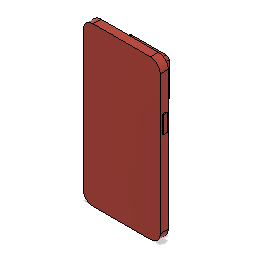
IPHONE_14Plus (PENDING CHECK) v4 (Autodesk Fusion 360 design; units mm, degrees)
Autodesk Fusion 360 part; units mm, degrees
sketch "Sketch1" plane through (0, 0, 0) normal (0, 0, 1) x (1, 0, 0)
  line L0 (39.05, 80.4) -> (-39.05, 80.4)
  line L1 (-39.05, 80.4) -> (-39.05, -80.4)
  line L2 (-39.05, -80.4) -> (39.05, -80.4)
  line L3 (39.05, -80.4) -> (39.05, 80.4)
  line L4 (39.05, 80.4) -> (-39.05, -80.4) construction
  line L5 (-39.05, 80.4) -> (39.05, -80.4) construction
  dimension "d1" = 78.1
  dimension "d2" = 160.8
  constraint horizontal L0
  constraint perpendicular L0 L1
  constraint parallel L0 L2
  constraint parallel L1 L3
  constraint coincident L4 origin
  constraint coincident L5 origin
  measures "d1" distance of L1.end L2.end
  measures "d2" distance of L0.end L1.end
extrude "Extrude1" add sketch "Sketch1" along normal blind 7.8 makes body 1
fillet "Fillet1" radius 10 4 edges at (-39.05, 80.4, 3.9) (39.05, 80.4, 3.9) (39.05, -80.4, 3.9) (-39.05, -80.4, 3.9) on bodies 1
sketch "Sketch3" plane through (0, 0, 0) normal (0, 0, -1) x (1, 0, 0)
  line L0 (-5.7, -37.375) -> (35.3, -37.375)
  line L1 (35.3, -37.375) -> (35.3, -77.375)
  line L2 (35.3, -77.375) -> (-5.7, -77.375)
  line L3 (-5.7, -77.375) -> (-5.7, -37.375)
  line L4 (-5.7, -37.375) -> (35.3, -77.375) construction
  line L5 (35.3, -37.375) -> (-5.7, -77.375) construction
  line L6 (-28.8, -80.375) -> (28.8, -80.375)
  line L7 (38.8, -70.375) -> (38.8, 70.375)
  arc A0 (-28.8, 80.375) -> (-38.8, 70.375) centre (-28.8, 70.375) ccw
  line L8 (-28.8, 80.375) -> (28.8, 80.375)
  arc A1 (38.8, 70.375) -> (28.8, 80.375) centre (28.8, 70.375) ccw
  line L9 (38.8, 70.375) -> (38.8, -70.375)
  arc A2 (28.8, -80.375) -> (38.8, -70.375) centre (28.8, -70.375) ccw
  line L10 (28.8, -80.375) -> (-28.8, -80.375)
  arc A3 (-38.8, -70.375) -> (-28.8, -80.375) centre (-28.8, -70.375) ccw
  line L11 (-38.8, -70.375) -> (-38.8, 70.375)
  arc A4 (-29.05, 80.4) -> (-39.05, 70.4) centre (-29.05, 70.4) ccw
  line L12 (-39.05, 70.4) -> (-39.05, -70.4)
  arc A5 (-39.05, -70.4) -> (-29.05, -80.4) centre (-29.05, -70.4) ccw
  line L13 (-29.05, -80.4) -> (29.05, -80.4)
  arc A6 (29.05, -80.4) -> (39.05, -70.4) centre (29.05, -70.4) ccw
  line L14 (39.05, -70.4) -> (39.05, 70.4)
  arc A7 (39.05, 70.4) -> (29.05, 80.4) centre (29.05, 70.4) ccw
  line L15 (29.05, 80.4) -> (-29.05, 80.4)
  point P0 (14.8, -57.375)
  dimension "d9" = 41
  dimension "d10" = 40
  dimension "d18" = 3
  dimension "d19" = 3.5
  constraint horizontal L0
  constraint perpendicular L0 L1
  constraint parallel L0 L2
  constraint parallel L1 L3
  constraint coincident L4 P0
  constraint coincident L5 P0
  measures "d9" distance of L0.start L0.end
  measures "d10" distance of L0.start L2.end
  measures "d18" distance of L2 L6
  measures "d19" distance of L1 L9
extrude "Extrude2" add sketch "Sketch3" along normal blind 4.5 contours L0 L1 L2 L3 bodies 1
fillet "Fillet2" radius 3 4 edges at (35.3, 77.375, -2.25) (35.3, 37.375, -2.25) (-5.7, 77.375, -2.25) (-5.7, 37.375, -2.25) on bodies 1
sketch "Sketch4" plane through (39.05, 0, 0) normal (1, 0, 0) x (0, 0, -1)
  line L0 (-7.8, -70.4) -> (0, -70.4)
  line L1 (0, -70.4) -> (0, 70.4)
  line L2 (0, 70.4) -> (-7.8, 70.4)
  line L3 (-7.8, 70.4) -> (-7.8, -70.4)
  line L4 (4.5, 40.375) -> (4.5, 37.375)
  line L5 (4.5, 37.375) -> (0, 37.375)
  line L6 (4.5, 40.375) -> (4.5, 74.375)
  line L7 (4.5, 77.375) -> (4.5, 74.375)
  line L8 (0, 77.375) -> (4.5, 77.375)
  line L9 (-7.8, -80.4) -> (-7.8, -70.4)
  line L10 (0, -70.4) -> (0, -80.4)
  line L11 (0, -80.4) -> (-7.8, -80.4)
  line L12 (0, 37.375) -> (0, -70.4)
  line L13 (0, 80.4) -> (0, 77.375)
  line L14 (-7.8, 80.4) -> (0, 80.4)
  line L15 (-7.8, 70.4) -> (-7.8, 80.4)
  line L16 (-7.8, 70.4) -> (-7.8, -70.4)
  line L17 (-3.9, 70.4) -> (-3.9, -70.4) construction
  line L18 (-1.9, 16.2) -> (-5.9, 16.2)
  line L19 (-5.9, 16.2) -> (-5.9, 33.9)
  line L20 (-5.9, 33.9) -> (-1.9, 33.9)
  line L21 (-1.9, 33.9) -> (-1.9, 16.2)
  line L22 (-1.9, 16.2) -> (-5.9, 33.9) construction
  line L23 (-5.9, 16.2) -> (-1.9, 33.9) construction
  point P0 (-3.9, 25.05)
  dimension "d20" = 4
  dimension "d21" = 17.7
  dimension "d22" = 46.5
  constraint midpoint L2 L17.start
  constraint midpoint L0 L17.end
  constraint horizontal L18
  constraint perpendicular L18 L19
  constraint parallel L18 L20
  constraint parallel L19 L21
  constraint coincident L22 P0
  constraint coincident L23 P0
  constraint coincident L17 P0
  measures "d20" distance of L18.start L18.end
  measures "d21" distance of L18.start L20.end
  measures "d22" distance of L14 L20
extrude "Extrude3" add sketch "Sketch4" along normal blind 1 contours L18 L19 L20 L21 bodies 1
sketch "Sketch5" plane through (-39.05, 0, 0) normal (-1, 0, 0) x (0, 0, 1)
  line L0 (0, -70.4) -> (7.8, -70.4)
  line L1 (7.8, -70.4) -> (7.8, 70.4)
  line L2 (7.8, 70.4) -> (0, 70.4)
  line L3 (0, 70.4) -> (0, -70.4)
  line L4 (-4.5, 74.375) -> (-4.5, 77.375)
  line L5 (-4.5, 74.375) -> (-4.5, 40.375)
  line L6 (-4.5, 37.375) -> (-4.5, 40.375)
  line L7 (0, 37.375) -> (-4.5, 37.375)
  line L8 (-4.5, 77.375) -> (0, 77.375)
  line L9 (7.8, -80.4) -> (0, -80.4)
  line L10 (0, 77.375) -> (0, 80.4)
  line L11 (0, -70.4) -> (0, 37.375)
  line L12 (0, -80.4) -> (0, -70.4)
  line L13 (7.8, -70.4) -> (7.8, -80.4)
  line L14 (7.8, -70.4) -> (7.8, 70.4)
  line L15 (7.8, 80.4) -> (7.8, 70.4)
  line L16 (0, 80.4) -> (7.8, 80.4)
  line L17 (3.9, 70.4) -> (3.9, -70.4) construction
  line L18 (5.225, 30.45) -> (2.575, 30.45)
  line L19 (2.575, 30.45) -> (2.575, 41.65)
  line L20 (2.575, 41.65) -> (5.225, 41.65)
  line L21 (5.225, 41.65) -> (5.225, 30.45)
  line L22 (5.225, 30.45) -> (2.575, 41.65) construction
  line L23 (2.575, 30.45) -> (5.225, 41.65) construction
  line L24 (0, 28.95) -> (7.8, 28.95) construction
  line L25 (2.575, 27.45) -> (2.575, 16.25)
  line L26 (2.575, 16.25) -> (5.225, 16.25)
  line L27 (5.225, 27.45) -> (2.575, 27.45)
  line L28 (5.225, 16.25) -> (5.225, 27.45)
  point P0 (3.9, 36.05)
  dimension "d25" = 1.5
  dimension "d26" = 11.2
  dimension "d27" = 2.65
  dimension "d28" = 38.75
  constraint midpoint L2 L17.start
  constraint midpoint L0 L17.end
  constraint horizontal L18
  constraint perpendicular L18 L19
  constraint parallel L18 L20
  constraint parallel L19 L21
  constraint coincident L22 P0
  constraint coincident L23 P0
  constraint coincident L17 P0
  constraint coincident L11 L24.start
  constraint coincident L14 L24.end
  constraint perpendicular L14 L24
  constraint symmetric L18.start L24 L27.start
  constraint symmetric L18.end L24 L25.start
  constraint symmetric L19.end L24 L25.end
  constraint symmetric L20.end L24 L26.end
  measures "d25" distance of L18 L24
  measures "d26" distance of L18.start L20.end
  measures "d27" distance of L18.start L18.end
  measures "d28" distance of L16 L20
extrude "Extrude4" add sketch "Sketch5" along normal blind 1 contours L18 L19 L20 L21 | L25 L26 L27 L28 bodies 1
copy_body "CopyPasteBodies1" bodies 1 makes body 2
move_body "Move1" bodies 2 to x (1, 0, 0) y (0, 1, 0) z (0, 0, 1) at (0, 0, 0)
scale "Scale1" factors (1.006, 1.003, 1.04) about (-2.7, 37.375, 0) bodies 2
copy_body "CopyPasteBodies2" bodies 2 makes body 3
move_body "Move2" bodies 3 to x (-1, 0, 0) y (0, -1, 0) z (0, 0, 1) at (0.0744, -0.228, 0)
hidden bodies 1 3
equation "d25 = ( 3 / 2 ) * 1 mm"
named bodies: "IPHONE_14Plus", "IPHONE_14P", "IPHONE_14Plus_FIT", "IPHONE_14P_FIT", "IPHONE_14Plus_FIT REVERSED"
